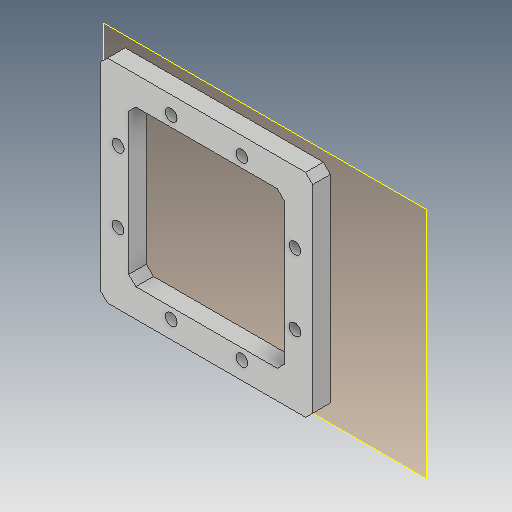
# Autodesk Inventor part: cellSTORM_UC2_spacer_XYstage
Saved by Autodesk Inventor 2019.4 (Build 234330000, 330)
## iProperties
Created: 2020-12-31
Part Number: cellSTORM_UC2_spacer_XYstage
Material: Generic
Document SubType Name: Modeling
Designer: diederichbenedict
Density: 1 g/cm^3
Appearance: Default
Author: diederichbenedict
Autodesk Inventor part; units mm, degrees
ref_plane "YZ Plane" through (0, 0, 0) normal (1, 0, 0) x (0, 1, 0)
ref_plane "XZ Plane" through (0, 0, 0) normal (0, 1, 0) x (-1, 0, 0)
ref_plane "XY Plane" through (0, 0, 0) normal (0, 0, 1) x (1, 0, 0)
ref_plane "Work Plane1" through (0, 0, 0) normal (0, 0, 1) x (1, 0, 0)
sketch "Sketch1" plane through (0, 0, 0) normal (0, 0, 1) x (1, 0, 0)
  line L0 (-12.7208, -13) -> (-12.7208, -2.8703) construction
  arc A0 (-12.7208, 0.8703) -> (-12.7208, -2.8703) centre (-15.6792, -1) ccw construction
  line L1 (-12.7208, 0.8703) -> (-12.7208, 19) construction
  line L2 (-12.7208, 19) -> (-62.6792, 19) construction
  line L3 (-62.6792, 19) -> (-62.6792, -12) construction
  line L4 (-62.6792, -12) -> (-70.6792, -12) construction
  line L5 (-70.6792, -12) -> (-70.6792, -41) construction
  line L6 (-70.6792, -41) -> (-10.6792, -41) construction
  line L7 (-10.6792, -41) -> (-10.6792, -19) construction
  line L8 (-10.6792, -19) -> (12.2792, -19) construction
  line L9 (12.2792, -19) -> (12.2792, 19) construction
  line L10 (12.2792, 19) -> (-7.7208, 19) construction
  line L11 (-7.7208, 19) -> (-7.7208, -13) construction
  line L12 (-7.7208, -13) -> (-12.7208, -13) construction
  circle A1 centre (2.2792, 3) radius 0.5 construction
  circle A2 centre (-50.6792, 14) radius 3.5 construction
  circle A3 centre (-30.6792, -36) radius 3.5 construction
  circle A4 centre (-50.6792, -36) radius 3.5 construction
  circle A5 centre (-15.6792, -21) radius 3.5 construction
  circle A6 centre (-30.6792, 14) radius 3.5 construction
  circle A7 centre (-65.6792, -21) radius 3.5 construction
  line L13 (-10.6792, -41) -> (-70.6792, -41)
  line L14 (-70.6792, -41) -> (-70.6792, 19)
  line L15 (-70.6792, 19) -> (-10.6792, 19)
  line L16 (-10.6792, 19) -> (-10.6792, -41)
  line L17 (-62.6792, -33) -> (-18.6792, -33)
  line L18 (-18.6792, -33) -> (-18.6792, 11)
  line L19 (-18.6792, 11) -> (-62.6792, 11)
  line L20 (-62.6792, 11) -> (-62.6792, -33)
  circle A8 centre (-15.6792, -21) radius 1.45 projected
  circle A9 centre (-15.6792, -1) radius 1.65 projected
  circle A10 centre (-30.6792, 14) radius 1.65 projected
  circle A11 centre (-50.6792, 14) radius 1.65 projected
  circle A12 centre (-50.6792, -36) radius 1.65 projected
  circle A13 centre (-30.6792, -36) radius 1.65 projected
  circle A14 centre (-15.6792, -21) radius 1.65 projected
  circle A15 centre (-65.6792, -21) radius 1.65 projected
  circle A16 centre (-65.6792, -1) radius 1.6945
  point P0 (0, 0)
  dimension "d0" = 8
  constraints: 16 end point, 4 parallel, 2 perpendicular, 1 centre point, 1 horizontal, 3 other
  measures "d0" distance between parallel lines of L13 L17
extrude "Extrusion1" add sketch "Sketch1" along normal blind 5 contours L13 L14 L15 L16
chamfer "Chamfer1" distance 2 angle 45 8 edges at (-10.6792, 19, 2.5) (-70.6792, 19, 2.5) (-10.6792, -41, 2.5) (-70.6792, -41, 2.5) (-18.6792, -33, 2.5) (-62.6792, -33, 2.5) (-18.6792, 11, 2.5) (-62.6792, 11, 2.5)
body "Solid1"
